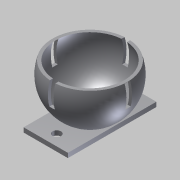
# Autodesk Inventor part: pingpongwheel2
Saved by Autodesk Inventor 2012 SP2 (Build 160219200, 219)
## iProperties
Created: 2015-01-08
Part Number: pingpongwheel2
Material: Default
Document SubType Name: Modeling
Designer: dahumphr
Density: 1 g/cm^3
Author: dahumphr
Autodesk Inventor part; units mm, degrees
note: some values were not read from the file. Chosen so that the rebuilt part matches the saved one: sketch regions of "Extrusion14".
sketch "Sketch1" plane through (0, 0, 0) normal (0, 0, 1) x (1, 0, 0)
  arc A0 (0, 20.955) -> (-19.7566, -6.985) centre (0, 0) ccw
  arc A1 (0, 22.606) -> (-21.4998, -6.985) centre (0, 0) ccw
  line L0 (0, 20.955) -> (0, 22.606)
  line L1 (0, 0) -> (0, -18.1078)
  line L2 (0, 22.606) -> (0, 20.955)
  line L3 (-29.2168, -6.985) -> (-5.4642, -6.985)
  dimension "d0" = 41.91
  dimension "d1" = 1.651
  dimension "d28" = 6.985
  constraints: 8 end point, 4 point on circle, 2 centre point, 2 coincident, 2 collinear, 2 point on line, 1 vertical
  measures "d0" diameter of A0
  measures "d1" radial gap between concentric circles of A0 A1
  measures "d28" distance from line of L3 point (0, 0)
ref_plane "Work Plane1" through (0, 21.6535, 0) normal (0, 1, 0) x (-1, 0, 0)
sketch "Sketch2" plane through (0, 21.6535, 0) normal (0, 1, 0) x (-1, 0, 0)
  circle A0 centre (0, 0) radius 21.6535 projected
  line L0 (-21.6535, 21.6535) -> (21.6535, 21.6535)
  line L1 (21.6535, 21.6535) -> (21.6535, -21.6535)
  line L2 (21.6535, -21.6535) -> (-21.6535, -21.6535)
  line L3 (-21.6535, -21.6535) -> (-21.6535, 21.6535)
  circle A1 centre (0, 0) radius 22.225
  dimension "d21" = 44.45
  constraints: 8 end point, 4 tangent, 2 parallel, 1 centre point, 1 coincident, 1 horizontal, 1 perpendicular
  measures "d21" diameter of A1
ref_plane "Work Plane4" through (21.6535, 18.4785, -21.6535) normal (0, 0, -1) x (-1, 0, 0)
sketch "Sketch5" plane through (21.6535, 18.4785, -21.6535) normal (0, 0, -1) x (-1, 0, 0)
  line L0 (43.307, 0) -> (0, 0) projected
  line L1 (20.066, -25.4159) -> (23.241, -25.4159)
  line L2 (23.241, -25.4159) -> (23.241, -12.577)
  line L3 (23.241, -12.577) -> (20.066, -12.577)
  line L4 (20.066, -12.577) -> (20.066, -25.4159)
  point P0 (21.6535, -18.4785)
  point P1 (21.6535, -12.577)
  point P2 (21.6535, 0)
  dimension "d8" = 3.175
  constraints: 8 end point, 2 midpoint, 2 parallel, 1 horizontal, 1 perpendicular, 1 vertical alignment
  measures "d8" distance of L3.end L2.end
ref_plane "Work Plane5" through (-21.6535, 18.4785, -21.6535) normal (-1, 0, 0) x (0, 0, 1)
sketch "Sketch6" plane through (-21.6535, 18.4785, -21.6535) normal (-1, 0, 0) x (0, 0, 1)
  line L0 (43.307, 0) -> (0, 0) projected
  line L1 (20.066, -12.577) -> (23.241, -12.577)
  line L2 (23.241, -12.577) -> (23.241, -25.5981)
  line L3 (23.241, -25.5981) -> (20.066, -25.5981)
  line L4 (20.066, -25.5981) -> (20.066, -12.577)
  line L5 (42.4873, -12.577) -> (42.4267, -12.577) projected
  point P0 (21.6535, -18.4785)
  point P1 (40.6996, -12.577)
  point P2 (21.6535, -12.577)
  point P3 (21.6535, 0)
  dimension "d11" = 3.175
  constraints: 8 end point, 2 midpoint, 2 parallel, 1 horizontal, 1 horizontal alignment, 1 perpendicular, 1 vertical alignment
  measures "d11" distance of L2.end L3.end
revolve "Revolution2" add sketch "Sketch1" angle 360 about axis through (0, 0, 0) along (0, -1, 0)
extrude "Extrusion6" cut sketch "Sketch5" along normal through all both and the other way through all
extrude "Extrusion7" cut sketch "Sketch6" along normal through all both and the other way through all
ref_plane "Work Plane6" through (0, 22.606, 0) normal (0, 1, 0) x (-1, 0, 0)
sketch "Sketch7" plane through (0, 22.606, 0) normal (0, 1, 0) x (-1, 0, 0)
  arc A0 (-22.5502, -1.5875) -> (-22.5502, 1.5875) centre (0, 0) ccw projected
  circle A1 centre (0, 0) radius 22.606
  constraints: 1 centre point, 1 coincident, 1 concentric
loft "Loft1" add profiles "Sketch2", "Sketch7" contours A0 | L1 A1 L2 A0 | A0 L0 A1 L1 | L1 A1 | A0 L3 A1 L0 | L0 A1 | L2 A1 L3 A0 | L2 A1 | L3 A1 / all
sketch "Sketch8" plane through (0, 21.6535, 0) normal (0, -1, 0) x (1, 0, 0)
  circle A0 centre (0, 0) radius 5.0077 projected
extrude "Extrusion8" cut sketch "Sketch8" against normal blind 25.4
sketch "Sketch9" plane through (0, 21.6535, 0) normal (0, -1, 0) x (1, 0, 0)
  circle A0 centre (0, 0) radius 5.0077 projected
  circle A1 centre (0, 0) radius 22.225 projected
extrude "Extrusion9" add sketch "Sketch9" along normal blind 1.651
sketch "Sketch10" plane through (0, 22.606, 0) normal (0, 1, 0) x (1, 0, 0)
  circle A0 centre (0, 0) radius 5.0077 projected
extrude "Extrusion10" cut sketch "Sketch10" against normal blind 25.4
sketch "Sketch11" plane through (0, 22.606, 0) normal (0, 1, 0) x (1, 0, 0)
  circle A0 centre (0, 0) radius 5.0077 projected
  line L0 (-25.4, 22.225) -> (25.4, 22.225)
  line L1 (25.4, 22.225) -> (25.4, -22.225)
  line L2 (25.4, -22.225) -> (-25.4, -22.225)
  line L3 (-25.4, -22.225) -> (-25.4, 22.225)
  circle A1 centre (-19.05, 0) radius 2.3813
  circle A2 centre (19.05, 0) radius 2.3812
  line L4 (-19.05, 0) -> (19.05, 0)
  line L5 (19.05, 0) -> (19.05, 0)
  line L6 (-25.4, -12.7) -> (25.4, -12.7)
  line L7 (25.4, -12.7) -> (25.4, 12.7)
  line L8 (25.4, 12.7) -> (-25.4, 12.7)
  line L9 (-25.4, 12.7) -> (-25.4, -12.7)
  point P0 (0, 22.225)
  point P1 (0, -7.1437)
  point P2 (25.4, 0)
  point P3 (-25.4, 0)
  point P4 (-25.4, 0)
  point P5 (25.4, 0)
  dimension "d33" = 50.8
  dimension "d34" = 4.7625
  dimension "d35" = 4.7625
  dimension "d36" = 38.1
  dimension "d49" = 25.4
  constraints: 20 end point, 7 midpoint, 4 coincident, 4 parallel, 3 perpendicular, 2 centre point, 2 horizontal, 2 horizontal alignment, 2 point on line, 1 vertical alignment
  measures "d33" distance of L0.start L0.end
  measures "d34" diameter of A1
  measures "d35" diameter of A2
  measures "d36" distance of L4.end L4.start
  measures "d49" distance between parallel lines of L6 L8
extrude "Extrusion14" cut sketch "Sketch11" against normal up to surface (2.6035 mm away) contours L0 L1 L8 L3 | L6 L1 L2 L3
extrude "Extrusion15" add sketch "Sketch11" against normal up to surface (2.6035 mm away) contours L8 L1 L6 L3
extrude "Extrusion16" cut sketch "Sketch11" against normal up to surface (2.6035 mm away) contours A1 | A2
sketch "Sketch14" plane through (-25.4, 22.606, 12.7) normal (0, 1, 0) x (1, 0, 0)
  line L0 (30.4077, 33.2343) -> (5.3772, 33.2343)
  line L1 (5.3772, 33.2343) -> (5.3772, 42.4419)
  line L2 (5.3772, 42.4419) -> (30.4077, 42.4419)
  line L3 (30.4077, 42.4419) -> (30.4077, 33.2343)
  line L4 (12.831, -6.0805) -> (37.6767, -6.0805)
  line L5 (37.6767, -6.0805) -> (37.6767, -14.7034)
  line L6 (37.6767, -14.7034) -> (12.831, -14.7034)
  line L7 (12.831, -14.7034) -> (12.831, -6.0805)
  constraints: 16 end point, 4 parallel, 2 horizontal, 2 perpendicular
extrude "Extrusion17" cut sketch "Sketch14" against normal up to surface (2.6035 mm away)
body "Solid1"
